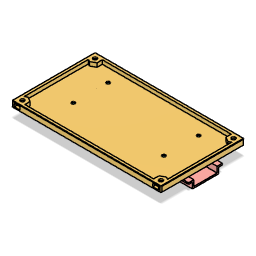
RelayBoardMount (Autodesk Fusion 360 design; units mm, degrees)
Autodesk Fusion 360 part; units mm, degrees
sketch "Skizze1" plane through (0, 0, 0) normal (1, 0, 0) x (0, 0, -1) in component "Rail"
  line L0 (-17.5, 0) -> (17.5, 0)
  line L1 (-13.5, -7.5) -> (13.5, -7.5)
  line L2 (0, -7.5) -> (0, 0) construction
  line L3 (-17.5, 0) -> (-17.5, -1.5)
  line L4 (17.5, 0) -> (17.5, -1.5)
  line L5 (13.5, -7.5) -> (13.5, -1.5)
  line L6 (13.5, -1.5) -> (17.5, -1.5)
  line L7 (-17.5, -1.5) -> (-13.5, -1.5)
  line L8 (-13.5, -1.5) -> (-13.5, -7.5)
  line L9 (-12, 0) -> (-12, -6)
  line L10 (-12, -6) -> (12, -6)
  line L11 (12, -6) -> (12, 0)
  dimension "d1" = 35
  dimension "d2" = 27
  dimension "d3" = 1.5
  dimension "d5" = 7.5
  dimension "d6" = 1.5
  dimension "d7" = 1.5
  dimension "d8" = 1.5
  constraint horizontal L0
  constraint midpoint L2.end L0
  constraint horizontal L1
  constraint midpoint L1 L2.start
  constraint coincident L2.end origin
  constraint vertical L2
  constraint perpendicular L0 L3
  constraint perpendicular L0 L4
  constraint perpendicular L1 L5
  constraint perpendicular L4 L6
  constraint perpendicular L5 L7
  constraint perpendicular L7 L8
  constraint equal L3 L4
  constraint coincident L0 L9.start
  constraint perpendicular L0 L9
  constraint perpendicular L5 L10
  constraint coincident L0 L11.end
  constraint perpendicular L0 L11
  measures "d1" distance of L0.start L0.end
  measures "d2" distance of L1.start L1.end
  measures "d3" distance of L0.end L4.end
  measures "d5" distance of L0 L1
  measures "d6" distance of L1 L10
  measures "d7" distance of L8 L9
  measures "d8" distance of L5 L11
extrude "Extrusion1" add sketch "Skizze1" along normal mid plane 160 contours L0 L1 L3 L4 L5 L6 L7 L8 L9 L10 L11 makes body 1 in component "Rail"
sketch "Skizze1 (2)" plane through (0, 0, 0) normal (0, 1, 0) x (1, 0, 0) in component "DinRailMount"
  line L0 (-80, 17.5) -> (80, 17.5)
  line L1 (-80, 12) -> (80, 12)
  line L2 (-80, -12) -> (80, -12)
  line L3 (80, -17.5) -> (-80, -17.5)
  line L4 (0, 17.5) -> (0, -17.5) construction
  line L5 (-5, 17.5) -> (5, 17.5)
  line L6 (5, 17.5) -> (5, 20.5)
  line L7 (5, 20.5) -> (-5, 20.5)
  line L8 (-5, 20.5) -> (-5, 17.5)
  arc A0 (0, 17.5) -> (0, 11.5) centre (0, 14.5) ccw
  arc A1 (0, 5.5) -> (0, 11.5) centre (0, 8.5) ccw
  arc A2 (0, 5.5) -> (0, -0.5) centre (0, 2.5) ccw
  arc A3 (0, -6.5) -> (0, -0.5) centre (0, -3.5) ccw
  arc A4 (0, -5.8) -> (0, -1.2) centre (0, -3.5) ccw
  arc A5 (0, 6.2) -> (0, -1.2) centre (0, 2.5) ccw
  arc A6 (0, 6.2) -> (0, 10.8) centre (0, 8.5) ccw
  arc A7 (0, 18.2) -> (0, 10.8) centre (0, 14.5) ccw
  arc A8 (0, 16.8) -> (0, 12.2) centre (0, 14.5) ccw
  arc A9 (0, 4.8) -> (0, 12.2) centre (0, 8.5) ccw
  arc A10 (0, 4.8) -> (0, 0.2) centre (0, 2.5) ccw
  arc A11 (0, -7.2) -> (0, 0.2) centre (0, -3.5) ccw
  arc A12 (0, 16.8) -> (5, 17.5) centre (0, 35.0071) ccw
  line L9 (-8.5, 22.5) -> (8.5, 22.5) construction
  line L10 (8.5, 22.5) -> (8.5, -20.5)
  line L11 (8.5, -20.5) -> (-8.5, -20.5)
  line L12 (-8.5, -20.5) -> (-8.5, 22.5)
  line L13 (0, -17.5) -> (0, -20.5) construction
  line L14 (-5.5, 22.5) -> (5.5, 22.5)
  line L15 (5.5, 22.5) -> (5.5, -6.5)
  line L16 (5.5, -6.5) -> (-5.5, -6.5)
  line L17 (-5.5, -6.5) -> (-5.5, 22.5)
  arc A13 (0, -5.8) -> (-5.5, -6.5) centre (0, -27.7571) ccw
  line L18 (8.5, 22.5) -> (8.5, 30.5)
  line L19 (8.5, 30.5) -> (-8.5, 30.5)
  line L20 (-8.5, 30.5) -> (-8.5, 22.5)
  line L21 (0, 30.5) -> (0, 22.5) construction
  circle A14 centre (0, 26.5) radius 1.75
  circle A15 centre (0, -9.5) radius 1.75
  dimension "d89" = 10
  dimension "d91" = 3
  dimension "d94" = 3
  dimension "d95" = 6
  dimension "d98" = 0
  dimension "d99" = -12
  dimension "d100" = 0.7
  dimension "d101" = -0.7
  dimension "d102" = 5
  dimension "d103" = 3
  dimension "d105" = 2
  dimension "d106" = 3.5
  dimension "d107" = 4
  dimension "d108" = 3
  dimension "d111" = 0.5
  dimension "d149" = 3
  constraint midpoint L0 L4.start
  constraint midpoint L3 L4.end
  constraint horizontal L5
  constraint vertical L6
  constraint horizontal L7
  constraint vertical L8
  constraint coincident L0 L5.start
  constraint midpoint L4.start L5
  constraint coincident L4 A0.end
  constraint coincident L4 A0.centre
  constraint coincident L4 A1.start
  constraint coincident L4 A1.centre
  constraint tangent A8 A12
  constraint horizontal L9
  constraint vertical L10
  constraint horizontal L11
  constraint vertical L12
  constraint midpoint L11 L13.end
  constraint collinear L4 L13
  constraint horizontal L14
  constraint vertical L15
  constraint horizontal L16
  constraint vertical L17
  constraint midpoint A3.start L16
  constraint tangent A4 A13
  constraint vertical L18
  constraint horizontal L19
  constraint vertical L20
  constraint coincident L9.end L10.start
  constraint midpoint L19 L21.start
  constraint midpoint L21 A14.centre
  constraint midpoint L14 L21.end
  constraint coincident L4 A15.centre
  constraint equal A14 A15
  measures "d89" distance of L5.start L5.end
  measures "d91" distance of L5.end L6.end
  measures "d94" distance of L5 A0.centre
  measures "d95" distance of A0.centre A1.centre
  measures "d102" distance of L0 L9
  measures "d103" distance of L3 L11
  measures "d105" distance of L7 L14
  measures "d106" diameter of A14
  measures "d107" distance of L19 A14.centre
  measures "d108" distance of L16 A15.centre
  measures "d111" distance of L8 L17
  measures "d149" distance of L12 L17
extrude "Extrusion1'" add sketch "Skizze1 (2)" along normal blind 3 separate body contours L0 L5 L6 L7 L8 | L0 L1 L5 A0 A7 | L0 L1 L5 A0 A8 A9 A12 | L1 A0 A1 A2 A3 A4 A5 A6 A7 L16 A13 | L1 A0 A1 A2 A3 A9 A10 A11 L16 | L0 L10 L12 L14 L15 L17 L18 L19 L20 | L0 L1 L10 L15 | L1 L2 L10 L12 L15 L16 L17 | L0 L1 L12 L17 | L2 L3 L10 L12 | L3 L10 L11 L12 makes body 2 in component "DinRailMount"
sketch "Skizze2" plane through (0, 3, 0) normal (0, 1, 0) x (-1, 0, 0) in component "DinRailMount"
  circle A0 centre (0, -26.5) radius 1.75
  circle A1 centre (0, 9.5) radius 1.75
  line L0 (5.5, 6.5) -> (5.5, -22.5)
  line L1 (5.5, -22.5) -> (-5.5, -22.5)
  line L2 (-5.5, -22.5) -> (-5.5, 6.5)
  line L3 (-5.5, 6.5) -> (-2.1656, 6.5)
  line L4 (-8.5, 20.5) -> (-8.5, -30.5)
  line L5 (-8.5, -30.5) -> (8.5, -30.5)
  line L6 (8.5, -30.5) -> (8.5, 20.5)
  line L7 (8.5, 20.5) -> (-8.5, 20.5)
  line L8 (5, -17.5) -> (6, -17.5)
  line L9 (6, -17.5) -> (6, -22)
  line L10 (6, -22) -> (5.5, -22)
  line L11 (5, -20.5) -> (6, -20.5)
  line L12 (5, -17) -> (6.5, -17)
  line L13 (6.5, -17) -> (6.5, -22.5)
  line L14 (6.5, -22.5) -> (5.5, -22.5)
  line L15 (-5, -17.5) -> (-6, -17.5)
  line L16 (-6, -17.5) -> (-6, -22)
  line L17 (-6, -22) -> (-5.5, -22)
  line L18 (-5, -20.5) -> (-6, -20.5)
  line L19 (-5, -17) -> (-6.5, -17)
  line L20 (-6.5, -17) -> (-6.5, -22.5)
  line L21 (-6.5, -22.5) -> (-5.5, -22.5)
  line L22 (5, -20.5) -> (5, -17.5)
  line L23 (5, -17.5) -> (2.1656, -17.5)
  line L24 (-5, -17.5) -> (-5, -20.5)
  line L25 (-5, -20.5) -> (5, -20.5)
  line L26 (-5, -17.5) -> (-5, -20.5)
  line L27 (-5, -20.5) -> (5, -20.5)
  line L28 (5, -20.5) -> (5, -17.5)
  line L29 (5, -17.5) -> (2.1656, -17.5)
  line L30 (-8.5, 20.5) -> (-8.5, -30.5)
  line L31 (-8.5, -30.5) -> (8.5, -30.5)
  line L32 (8.5, -30.5) -> (8.5, 20.5)
  line L33 (8.5, 20.5) -> (-8.5, 20.5)
  circle A2 centre (0, 9.5) radius 1.75
  circle A3 centre (0, -26.5) radius 1.75
  line L34 (5.5, 6.5) -> (5.5, -22.5)
  line L35 (5.5, -22.5) -> (-5.5, -22.5)
  line L36 (-5.5, -22.5) -> (-5.5, 6.5)
  line L37 (-5.5, 6.5) -> (-2.1656, 6.5)
  arc A4 (0, -4.8) -> (0, -12.2) centre (0, -8.5) ccw
  arc A5 (0, -16.8) -> (0, -12.2) centre (0, -14.5) ccw
  arc A6 (0, -16.8) -> (-5, -17.5) centre (0, -35.0071) ccw
  arc A7 (2.1656, -17.5) -> (0, -10.8) centre (0, -14.5) ccw
  arc A8 (0, -6.2) -> (0, -10.8) centre (0, -8.5) ccw
  arc A9 (0, -6.2) -> (0, 1.2) centre (0, -2.5) ccw
  arc A10 (0, 5.8) -> (0, 1.2) centre (0, 3.5) ccw
  arc A11 (0, 5.8) -> (5.5, 6.5) centre (0, 27.7571) ccw
  arc A12 (-2.1656, 6.5) -> (0, -0.2) centre (0, 3.5) ccw
  arc A13 (0, -4.8) -> (0, -0.2) centre (0, -2.5) ccw
  arc A14 (0, -4.8) -> (0, -12.2) centre (0, -8.5) ccw
  arc A15 (0, -16.8) -> (0, -12.2) centre (0, -14.5) ccw
  arc A16 (0, -16.8) -> (-5, -17.5) centre (0, -35.0071) ccw
  arc A17 (2.1656, -17.5) -> (0, -10.8) centre (0, -14.5) ccw
  arc A18 (0, -6.2) -> (0, -10.8) centre (0, -8.5) ccw
  arc A19 (0, -6.2) -> (0, 1.2) centre (0, -2.5) ccw
  arc A20 (0, 5.8) -> (0, 1.2) centre (0, 3.5) ccw
  arc A21 (0, 5.8) -> (5.5, 6.5) centre (0, 27.7571) ccw
  arc A22 (-2.1656, 6.5) -> (0, -0.2) centre (0, 3.5) ccw
  arc A23 (0, -4.8) -> (0, -0.2) centre (0, -2.5) ccw
  dimension "d119" = 0.5
  dimension "d120" = -0.5
  dimension "d121" = 0.5
  dimension "d148" = 0.5
  constraint perpendicular L1 L9
  constraint perpendicular L0 L10
  constraint coincident L9 L11.end
  constraint perpendicular L9 L11
  constraint coincident L0 L10.end
  constraint coincident L1 L0.end
  constraint perpendicular L2 L15
  constraint perpendicular L15 L16
  constraint coincident L2 L17.end
  constraint perpendicular L2 L17
  constraint coincident L16 L18.end
  constraint perpendicular L16 L18
  constraint equal L8 L15
  constraint equal L9 L16
  measures "d119" distance of L0 L9
  measures "d121" distance of L1 L10
extrude "Extrusion2" cut sketch "Skizze2" against normal blind 1.4 from surface at -0.5 contours L0 L8 L9 L10 L12 L13 L14 L34 | L0 L9 L10 L11 L34 | L0 L8 L9 L11 L34 | L2 L15 L16 L17 L19 L20 L21 L36 | L2 L16 L17 L18 L36 | L2 L15 L16 L18 L36 bodies 2 in component "DinRailMount"
extrude "Extrusion3" add sketch "Skizze2" along normal blind 1 from surface at -1.7 contours L0 L8 L11 L22 L28 L34 | L0 L8 L9 L11 L34 | L2 L15 L18 L24 L26 L36 | L2 L15 L16 L18 L36 bodies 2 in component "DinRailMount"
sketch "Skizze3" plane through (5, 0, 0) normal (1, 0, 0) x (0, 0, -1) in component "DinRailMount"
  line L0 (20.5, 1.3) -> (17.5, 1.3)
  line L1 (17.5, 0) -> (20.5, 0)
  line L2 (20.5, 0) -> (20.5, 1.3)
  line L3 (-17.5, 0) -> (-17.5, -1.5)
  line L4 (-17.5, -1.5) -> (-13.5, -1.5)
  line L5 (-13.5, -1.5) -> (-13.5, -7.5)
  line L6 (-13.5, -7.5) -> (13.5, -7.5)
  line L7 (13.5, -7.5) -> (13.5, -1.5)
  line L8 (13.5, -1.5) -> (17.5, -1.5)
  line L9 (17.5, -1.5) -> (17.5, 0)
  line L10 (17.5, 0) -> (12, 0)
  line L11 (12, 0) -> (12, -6)
  line L12 (12, -6) -> (-12, -6)
  line L13 (-12, -6) -> (-12, 0)
  line L14 (-12, 0) -> (-17.5, 0)
  line L15 (20.5, 0) -> (20.5, -2)
  line L16 (16, -2) -> (16, -1.5)
  line L17 (16, -2) -> (17, -3)
  line L18 (17, -3) -> (19.5, -3)
  line L19 (19.5, -3) -> (20.5, -2)
  line L20 (20.5, -2) -> (16, -2) construction
  line L21 (17.5, 1.3) -> (17.5, 0)
  dimension "d127" = 1.5
  dimension "d129" = 0.5
  dimension "d130" = 1.5
  dimension "d151" = 45
  dimension "d152" = 45
  constraint coincident L1.end L2.start
  constraint perpendicular L1 L15
  constraint coincident L8 L16.end
  constraint perpendicular L8 L16
  constraint horizontal L18
  constraint perpendicular L16 L20
  measures "d127" distance of L9 L16
  measures "d129" distance of L16.start L16.end
  measures "d130" distance of L8 L18
  measures "d151" angle of L17 L20
  measures "d152" angle of L19 L20
extrude "Extrusion4" add sketch "Skizze3" against normal up to surface (10 mm away) contours L1 L8 L9 L15 L16 L17 L18 L19 bodies 2 in component "DinRailMount"
sketch "Skizze4" plane through (8.5, 0, 0) normal (1, 0, 0) x (0, 0, -1) in component "DinRailMount"
  line L0 (-20.5, 0) -> (30.5, 0)
  line L1 (30.5, 0) -> (30.5, 3)
  line L2 (30.5, 3) -> (-20.5, 3)
  line L3 (-20.5, 3) -> (-20.5, 0)
  line L4 (-17.5, 0) -> (-17.5, -1.5)
  line L5 (-17.5, -1.5) -> (-13.5, -1.5)
  line L6 (-13.5, -1.5) -> (-13.5, -7.5)
  line L7 (-13.5, -7.5) -> (13.5, -7.5)
  line L8 (13.5, -7.5) -> (13.5, -1.5)
  line L9 (13.5, -1.5) -> (17.5, -1.5)
  line L10 (17.5, -1.5) -> (17.5, 0)
  line L11 (17.5, 0) -> (12, 0)
  line L12 (12, 0) -> (12, -6)
  line L13 (12, -6) -> (-12, -6)
  line L14 (-12, -6) -> (-12, 0)
  line L15 (-12, 0) -> (-17.5, 0)
  line L16 (-20.5, 0) -> (-20.5, -2)
  line L17 (-19.5, -3) -> (-20.5, -2)
  line L18 (-17, -3) -> (-19.5, -3)
  line L19 (-16, -2) -> (-17, -3)
  line L20 (-16, -2) -> (-16, -1.5)
  line L21 (-16, -2) -> (-20.5, -2) construction
  dimension "d141" = 0.5
  dimension "d143" = 1.5
  dimension "d144" = 1.5
  dimension "d153" = 45
  dimension "d154" = 45
  constraint coincident L0 L3.end
  constraint coincident L0.start L3.end
  constraint coincident L5 L20.end
  constraint perpendicular L5 L20
  constraint perpendicular L0 L16
  constraint perpendicular L20 L21
  measures "d141" distance of L19.start L20.end
  measures "d143" distance of L5 L18
  measures "d144" distance of L4 L20
  measures "d153" angle of L17 L21
  measures "d154" angle of L19 L21
extrude "Extrusion5" add sketch "Skizze4" against normal up to surface (17 mm away) contours L0 L4 L5 L16 L17 L18 L19 L20 bodies 2 in component "DinRailMount"
chamfer "Fase1" distance 1 angle 45 2 edges at (-1.6316, 0, -27.1328) (-1.6316, 0, 8.8672) on bodies 2 in component "DinRailMount"
ref_plane "Arbeitsebene1" through (0, 2, -5) normal (0, 1, 0) x (1, 0, 0) in component "DinRailMount"
sketch "Skizze2 (2)" plane through (0, 2, 0) normal (0, 1, 0) x (1, 0, 0) in component "RelayBottom"
  line L0 (-74, 40) -> (74, 40)
  line L1 (74, 40) -> (74, -40)
  line L2 (74, -40) -> (-74, -40)
  line L3 (-74, -40) -> (-74, 40)
  line L4 (-74, 40) -> (74, -40) construction
  line L5 (74, 40) -> (-74, -40) construction
  line L6 (-77, 43) -> (77, 43)
  line L7 (77, 43) -> (77, -43)
  line L8 (77, -43) -> (-77, -43)
  line L9 (-77, -43) -> (-77, 43)
  circle A0 centre (-71.5, 37.5) radius 2
  line L10 (71.5, -37.5) -> (-71.5, -37.5) construction
  line L11 (-71.5, -37.5) -> (-71.5, 37.5) construction
  line L12 (-71.5, 37.5) -> (71.5, 37.5) construction
  line L13 (71.5, 37.5) -> (71.5, -37.5) construction
  line L14 (71.5, -37.5) -> (-71.5, 37.5) construction
  line L15 (-71.5, -37.5) -> (71.5, 37.5) construction
  circle A1 centre (71.5, 37.5) radius 2
  circle A2 centre (71.5, -37.5) radius 2
  circle A3 centre (-71.5, -37.5) radius 2
  line L16 (-68.5, 39.2321) -> (-71.5, 40.9641)
  line L17 (-71.5, 40.9641) -> (-74.5, 39.2321)
  line L18 (-74.5, 39.2321) -> (-74.5, 35.7679)
  line L19 (-74.5, 35.7679) -> (-71.5, 34.0359)
  line L20 (-71.5, 34.0359) -> (-68.5, 35.7679)
  line L21 (-68.5, 35.7679) -> (-68.5, 39.2321)
  line L22 (-68.5, 39.2321) -> (-68.5, 43)
  line L23 (-74.5, 39.2321) -> (-74.5, 43)
  line L24 (74.5, 35.7679) -> (74.5, 39.2321)
  line L25 (74.5, 39.2321) -> (71.5, 40.9641)
  line L26 (71.5, 40.9641) -> (68.5, 39.2321)
  line L27 (68.5, 39.2321) -> (68.5, 35.7679)
  line L28 (68.5, 35.7679) -> (71.5, 34.0359)
  line L29 (71.5, 34.0359) -> (74.5, 35.7679)
  line L30 (74.5, -35.7679) -> (71.5, -34.0359)
  line L31 (71.5, -34.0359) -> (68.5, -35.7679)
  line L32 (68.5, -35.7679) -> (68.5, -39.2321)
  line L33 (68.5, -39.2321) -> (71.5, -40.9641)
  line L34 (71.5, -40.9641) -> (74.5, -39.2321)
  line L35 (74.5, -39.2321) -> (74.5, -35.7679)
  line L36 (-68.5, -35.7679) -> (-71.5, -34.0359)
  line L37 (-71.5, -34.0359) -> (-74.5, -35.7679)
  line L38 (-74.5, -35.7679) -> (-74.5, -39.2321)
  line L39 (-74.5, -39.2321) -> (-71.5, -40.9641)
  line L40 (-71.5, -40.9641) -> (-68.5, -39.2321)
  line L41 (-68.5, -39.2321) -> (-68.5, -35.7679)
  line L42 (-74.5, -39.2321) -> (-74.5, -43)
  line L43 (-68.5, -39.2321) -> (-68.5, -43)
  line L44 (68.5, -39.2321) -> (68.5, -43)
  line L45 (74.5, -39.2321) -> (74.5, -43)
  line L46 (68.5, 39.2321) -> (68.5, 43)
  line L47 (74.5, 39.2321) -> (74.5, 43)
  line L48 (66.5, -39.2321) -> (66.5, -43)
  line L49 (66.5, -34.6132) -> (66.5, -39.2321)
  line L50 (71.5, -31.7265) -> (66.5, -34.6132)
  line L51 (76.5, -34.6132) -> (71.5, -31.7265)
  line L52 (76.5, -39.2321) -> (76.5, -34.6132)
  line L53 (76.5, -39.2321) -> (76.5, -43)
  line L54 (76.5, 39.2321) -> (76.5, 43)
  line L55 (76.5, 34.6132) -> (76.5, 39.2321)
  line L56 (71.5, 31.7265) -> (76.5, 34.6132)
  line L57 (66.5, 34.6132) -> (71.5, 31.7265)
  line L58 (66.5, 39.2321) -> (66.5, 34.6132)
  line L59 (66.5, 39.2321) -> (66.5, 43)
  line L60 (-66.5, 39.2321) -> (-66.5, 43)
  line L61 (-66.5, 34.6132) -> (-66.5, 39.2321)
  line L62 (-71.5, 31.7265) -> (-66.5, 34.6132)
  line L63 (-76.5, 34.6132) -> (-71.5, 31.7265)
  line L64 (-76.5, 39.2321) -> (-76.5, 34.6132)
  line L65 (-76.5, 39.2321) -> (-76.5, 43)
  line L66 (-76.5, -39.2321) -> (-76.5, -43)
  line L67 (-76.5, -34.6132) -> (-76.5, -39.2321)
  line L68 (-71.5, -31.7265) -> (-76.5, -34.6132)
  line L69 (-66.5, -34.6132) -> (-71.5, -31.7265)
  line L70 (-66.5, -39.2321) -> (-66.5, -34.6132)
  line L71 (-66.5, -39.2321) -> (-66.5, -43)
  point P0 (-71.5, 37.5)
  point P1 (71.5, 37.5)
  point P2 (71.5, -37.5)
  point P3 (-71.5, -37.5)
  dimension "d21" = 148
  dimension "d22" = 80
  dimension "d23" = -3
  dimension "d26" = 4
  dimension "d28" = 2.5
  dimension "d29" = 2.5
  dimension "d31" = 6
  dimension "d35" = 2
  dimension "d36" = 2
  dimension "d37" = -2
  dimension "d38" = 2
  constraint horizontal L0
  constraint perpendicular L0 L1
  constraint parallel L0 L2
  constraint parallel L1 L3
  constraint coincident L4 origin
  constraint coincident L5 origin
  constraint horizontal L10
  constraint perpendicular L10 L11
  constraint parallel L10 L12
  constraint parallel L11 L13
  constraint coincident L14 origin
  constraint coincident L15 origin
  constraint coincident P0 A0.centre
  constraint coincident P1 L12.end
  constraint coincident P2 L10.start
  constraint coincident P3 L10.end
  constraint equal A0 A3
  constraint equal A0 A2
  constraint equal A0 A1
  constraint coincident L6 L22.end
  constraint perpendicular L6 L22
  constraint coincident L6 L23.end
  constraint perpendicular L6 L23
  constraint collinear L21 L22
  constraint equal L21 L26
  constraint equal L21 L32
  constraint equal L21 L41
  constraint coincident L8 L42.end
  constraint parallel L38 L42
  constraint perpendicular L8 L42
  constraint coincident L8 L43.end
  constraint perpendicular L8 L43
  constraint coincident L8 L44.end
  constraint perpendicular L8 L44
  constraint collinear L32 L44
  constraint coincident L8 L45.end
  constraint perpendicular L8 L45
  constraint coincident L6 L46.end
  constraint perpendicular L6 L46
  constraint collinear L27 L46
  constraint coincident L6 L47.end
  constraint perpendicular L6 L47
  measures "d21" distance of L1.end L2.end
  measures "d22" distance of L0.end L1.end
  measures "d26" diameter of A0
  measures "d28" distance of L1 L13
  measures "d29" distance of L2 L10
  measures "d31" distance of L18 L21
extrude "Extrusion2'" add sketch "Skizze2 (2)" along normal blind 2 separate body contours L0 L3 L6 L16 L17 L22 L23 | L0 L3 L17 | L0 L16 L17 | L0 L3 L16 L17 L19 L20 L21 | L3 L17 L18 L19 | L0 L16 L22 | L0 L3 L19 L20 L21 L22 L60 L61 L62 L63 | L3 L6 L18 L19 L23 L63 L64 L65 | L0 L6 L22 L60 | L0 L1 L2 L3 L48 L49 L50 L51 L56 L57 L58 L59 L60 L61 L62 L63 L68 L69 L70 L71 | L3 L6 L8 L9 L63 L64 L65 L66 L67 L68 | L0 L6 L59 L60 | L2 L3 L36 L37 L41 L43 L68 L69 L70 L71 | L3 L8 L37 L38 L42 L66 L67 L68 | L0 L6 L46 L59 | L0 L1 L27 L28 L29 L46 L56 L57 L58 L59 | L2 L3 L36 L37 L39 L40 L41 | L3 L37 L38 L39 | L0 L1 L6 L25 L26 L46 L47 | L0 L26 L46 | L2 L3 L39 | L2 L3 L8 L39 L40 L42 L43 | L0 L25 L26 | L0 L1 L25 L26 L27 L28 L29 | L2 L39 L40 | L0 L1 L25 | L1 L6 L24 L29 L47 L54 L55 L56 | L2 L40 L43 | L2 L8 L43 L71 | L2 L8 L48 L71 | L1 L24 L25 L29 | L1 L6 L7 L8 L51 L52 L53 L54 L55 L56 | L1 L2 L30 L31 L32 L44 L48 L49 L50 L51 | L2 L8 L44 L48 | L1 L8 L30 L35 L45 L51 L52 L53 | L2 L33 L44 | L1 L2 L8 L33 L34 L44 L45 | L1 L30 L34 L35 | L1 L2 L30 L31 L32 L33 L34 | L2 L33 L34 | L1 L2 L34 | A0 | A1 | A2 | A3 makes body 3 in component "RelayBottom"
extrude "Extrusion4'" add sketch "Skizze2 (2)" along normal blind 4 from surface at 2 contours L0 L3 L6 L16 L17 L22 L23 | L0 L3 L17 | L0 L16 L17 | L0 L3 L16 L17 L19 L20 L21 | L3 L17 L18 L19 | L0 L16 L22 | L0 L3 L19 L20 L21 L22 L60 L61 L62 L63 | L3 L6 L18 L19 L23 L63 L64 L65 | L0 L6 L22 L60 | L3 L6 L8 L9 L63 L64 L65 L66 L67 L68 | L0 L6 L59 L60 | L2 L3 L36 L37 L41 L43 L68 L69 L70 L71 | L3 L8 L37 L38 L42 L66 L67 L68 | L0 L6 L46 L59 | L0 L1 L27 L28 L29 L46 L56 L57 L58 L59 | L2 L3 L36 L37 L39 L40 L41 | L3 L37 L38 L39 | L0 L1 L6 L25 L26 L46 L47 | L0 L26 L46 | L2 L3 L39 | L2 L3 L8 L39 L40 L42 L43 | L0 L25 L26 | L0 L1 L25 L26 L27 L28 L29 | L2 L39 L40 | L0 L1 L25 | L1 L6 L24 L29 L47 L54 L55 L56 | L2 L40 L43 | L2 L8 L43 L71 | L2 L8 L48 L71 | L1 L24 L25 L29 | L1 L6 L7 L8 L51 L52 L53 L54 L55 L56 | L1 L2 L30 L31 L32 L44 L48 L49 L50 L51 | L2 L8 L44 L48 | L1 L8 L30 L35 L45 L51 L52 L53 | L2 L33 L44 | L1 L2 L8 L33 L34 L44 L45 | L1 L30 L34 L35 | L1 L2 L30 L31 L32 L33 L34 | L2 L33 L34 | L1 L2 L34 bodies 3 in component "RelayBottom"
extrude "Extrusion3'" cut sketch "Skizze2 (2)" along normal blind 3 from surface at 1.5 contours L0 L3 L6 L16 L17 L22 L23 | L0 L3 L17 | L0 L16 L17 | L0 L3 L16 L17 L19 L20 L21 | L3 L17 L18 L19 | L0 L16 L22 | L2 L3 L36 L37 L39 L40 L41 | L3 L37 L38 L39 | L0 L1 L6 L25 L26 L46 L47 | L0 L26 L46 | L2 L3 L39 | L2 L3 L8 L39 L40 L42 L43 | L0 L25 L26 | L0 L1 L25 L26 L27 L28 L29 | L2 L39 L40 | L0 L1 L25 | L2 L40 L43 | L1 L24 L25 L29 | L2 L33 L44 | L1 L2 L8 L33 L34 L44 L45 | L1 L30 L34 L35 | L1 L2 L30 L31 L32 L33 L34 | L2 L33 L34 | L1 L2 L34 | A0 | A1 | A2 | A3 bodies 3 in component "RelayBottom"
sketch "Skizze4 (2)" plane through (0, 2, 0) normal (0, -1, 0) x (1, 0, 0) in component "RelayBottom"
  line L0 (77, 43) -> (-77, 43)
  line L1 (-77, 43) -> (-77, -43)
  line L2 (-77, -43) -> (77, -43)
  line L3 (77, -43) -> (77, 43)
  line L4 (-77, 0) -> (-47, 0) construction
  line L5 (77, 0) -> (47, 0) construction
  dimension "d158" = 30
  constraint midpoint L1 L4.start
  constraint perpendicular L1 L4
  constraint midpoint L3 L5.start
  constraint perpendicular L3 L5
  constraint equal L4 L5
  measures "d158" distance of L4.start L4.end
sketch "Skizze5" plane through (0, 2, 0) normal (0, -1, 0) x (1, 0, 0) in component "RelayBottom"
  line L0 (77, 43) -> (-77, 43)
  line L1 (-77, 43) -> (-77, -43)
  line L2 (-77, -43) -> (77, -43)
  line L3 (77, -43) -> (77, 43)
  line L4 (-41.5, 6.5) -> (-44.8344, 6.5)
  line L5 (-52.5, 6.5) -> (-52.5, -22.5)
  line L6 (-52.5, -22.5) -> (-41.5, -22.5)
  line L7 (-41.5, -22.5) -> (-41.5, 6.5)
  circle A0 centre (-47, -26.5) radius 1.75
  circle A1 centre (-47, 9.5) radius 1.75
  line L8 (-38.5, 20.5) -> (-38.5, -30.5)
  line L9 (-38.5, -30.5) -> (-55.5, -30.5)
  line L10 (-55.5, -30.5) -> (-55.5, 20.5)
  line L11 (-55.5, 20.5) -> (-38.5, 20.5)
  line L12 (52.5, 7) -> (49.1656, 7)
  line L13 (41.5, 7) -> (41.5, -22)
  line L14 (41.5, -22) -> (52.5, -22)
  line L15 (52.5, -22) -> (52.5, 7)
  circle A2 centre (47, -26) radius 1.75
  circle A3 centre (47, 10) radius 1.75
  line L16 (55.5, 21) -> (55.5, -30)
  line L17 (55.5, -30) -> (38.5, -30)
  line L18 (38.5, -30) -> (38.5, 21)
  line L19 (38.5, 21) -> (55.5, 21)
  line L20 (-38.1, -30.9) -> (-55.9, -30.9)
  line L21 (-55.9, -30.9) -> (-55.9, 20.9)
  line L22 (-55.9, 20.9) -> (-38.1, 20.9)
  line L23 (-38.1, 20.9) -> (-38.1, -30.9)
  line L24 (55.9, -30.4) -> (38.1, -30.4)
  line L25 (38.1, -30.4) -> (38.1, 21.4)
  line L26 (38.1, 21.4) -> (55.9, 21.4)
  line L27 (55.9, 21.4) -> (55.9, -30.4)
  line L28 (-42, -17.5) -> (-42, -20.5)
  line L29 (-42, -20.5) -> (-52, -20.5)
  line L30 (-52, -20.5) -> (-52, -17.5)
  line L31 (-52, -17.5) -> (-49.1656, -17.5)
  line L32 (52, -17) -> (52, -20)
  line L33 (52, -20) -> (42, -20)
  line L34 (42, -20) -> (42, -17)
  line L35 (42, -17) -> (44.8344, -17)
  arc A4 (-47, -10.8) -> (-47, -6.2) centre (-47, -8.5) ccw
  arc A5 (-47, 1.2) -> (-47, -6.2) centre (-47, -2.5) ccw
  arc A6 (-47, 1.2) -> (-47, 5.8) centre (-47, 3.5) ccw
  arc A7 (-52.5, 6.5) -> (-47, 5.8) centre (-47, 27.7571) ccw
  arc A8 (-47, -0.2) -> (-44.8344, 6.5) centre (-47, 3.5) ccw
  arc A9 (-47, -0.2) -> (-47, -4.8) centre (-47, -2.5) ccw
  arc A10 (-47, -12.2) -> (-47, -4.8) centre (-47, -8.5) ccw
  arc A11 (-47, -12.2) -> (-47, -16.8) centre (-47, -14.5) ccw
  arc A12 (-42, -17.5) -> (-47, -16.8) centre (-47, -35.0071) ccw
  arc A13 (-47, -10.8) -> (-49.1656, -17.5) centre (-47, -14.5) ccw
  arc A14 (47, -10.3) -> (47, -5.7) centre (47, -8) ccw
  arc A15 (47, 1.7) -> (47, -5.7) centre (47, -2) ccw
  arc A16 (47, 1.7) -> (47, 6.3) centre (47, 4) ccw
  arc A17 (41.5, 7) -> (47, 6.3) centre (47, 28.2571) ccw
  arc A18 (47, 0.3) -> (49.1656, 7) centre (47, 4) ccw
  arc A19 (47, 0.3) -> (47, -4.3) centre (47, -2) ccw
  arc A20 (47, -11.7) -> (47, -4.3) centre (47, -8) ccw
  arc A21 (47, -11.7) -> (47, -16.3) centre (47, -14) ccw
  arc A22 (52, -17) -> (47, -16.3) centre (47, -34.5071) ccw
  arc A23 (47, -10.3) -> (44.8344, -17) centre (47, -14) ccw
  dimension "d159" = -0.4
  dimension "d160" = -0.4
extrude "Extrusion8" cut sketch "Skizze5" against normal blind 1 contours L4 L5 L6 L7 L28 L29 L30 L31 A4 A5 A6 A7 A8 A9 A10 A11 A12 A13 | A0 | A1 | L8 L9 L10 L11 | L12 L13 L14 L15 L32 L33 L34 L35 A14 A15 A16 A17 A18 A19 A20 A21 A22 A23 | A2 | A3 | L16 L17 L18 L19 | L20 L21 L22 L23 | L24 L25 L26 L27 bodies 3 in component "RelayBottom"
extrude "Extrusion9" cut sketch "Skizze5" against normal up to surface (2 mm away) contours A0 | A1 | A2 | A3 bodies 3 in component "RelayBottom"
fillet "Abrundung2" radius 1 4 edges at (-77, 5, 43) (77, 5, 43) (77, 5, -43) (-77, 5, -43) on bodies 3 in component "RelayBottom"
chamfer "Fase3" distance 0.4 angle 45 16 edges at (0, 2, -43) (76.7071, 2, -42.7071) (77, 2, 0) (76.7071, 2, 42.7071) (0, 2, 43) (-76.7071, 2, 42.7071) (-77, 2, 0) (-76.7071, 2, -42.7071) (0, 8, -43) (-76.7071, 8, -42.7071) (-77, 8, 0) (-76.7071, 8, 42.7071) (0, 8, 43) (76.7071, 8, 42.7071) (77, 8, 0) (76.7071, 8, -42.7071) on bodies 3 in component "RelayBottom"
chamfer "Fase3" distance 0.4 angle 45 8 edges at (-38.1, 2, -5) (-47, 2, 20.9) (-55.9, 2, -5) (-47, 2, -30.9) (55.9, 2, -4.5) (47, 2, 21.4) (38.1, 2, -4.5) (47, 2, -30.4) on bodies 3 in component "RelayBottom"
component "Rail" placed x (1, 0, 0) y (0, 1, 0) z (0, 0, 1) at (0, 0, 0)
component "DinRailMount" placed x (1, 0, 0) y (0, 1, 0) z (0, 0, 1) at (-47, 0, 0)
component "DinRailMount" placed x (1, 0, 0) y (0, 1, 0) z (0, 0, 1) at (47, 0, 0.5)
component "RelayBottom" placed x (1, 0, 0) y (0, 1, 0) z (0, 0, 1) at (0, 0, 0)
